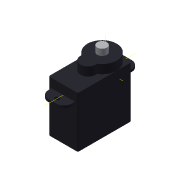
# Autodesk Inventor part: empty
Saved by Autodesk Inventor 2014 (Build 180170000, 170)
## iProperties
Created: 2015-04-13
Part Number: empty
Material: Generic
Document SubType Name: Modeling
Designer: Martin
Density: 1 g/cm^3
Appearance: Default
Author: Martin
Autodesk Inventor part; units mm, degrees
ref_plane "YZ Plane" through (0, 0, 0) normal (1, 0, 0) x (0, 1, 0)
ref_plane "XZ Plane" through (0, 0, 0) normal (0, 1, 0) x (-1, 0, 0)
ref_plane "XY Plane" through (0, 0, 0) normal (0, 0, 1) x (1, 0, 0)
sketch "Sketch1" plane through (0, 0, 0) normal (1, 0, 0) x (0, 1, 0)
  line L0 (0, -20.5) -> (0, 7.5) projected
  line L1 (-20.7, 0) -> (8.7, 0) projected
  line L2 (4.5, 3.5) -> (-16.5, 3.5)
  line L3 (-16.5, 3.5) -> (-16.5, -16.5)
  line L4 (-16.5, -16.5) -> (4.5, -16.5)
  line L5 (4.5, -16.5) -> (4.5, 3.5)
  point P0 (0, 0)
  dimension "d0" = 4.5
  dimension "d1" = 20
  dimension "d2" = 21
  dimension "d3" = 3.5
  constraints: 8 end point, 2 parallel, 1 horizontal, 1 perpendicular
  measures "d0" distance between parallel lines of L5 L0
  measures "d1" distance of L4.end L2.start
  measures "d2" distance of L3.end L4.end
  measures "d3" distance between parallel lines of L1 L2
extrude "Extrusion1" add sketch "Sketch1" along normal mid plane 11.5
sketch "Sketch2" plane through (0, 0, 0) normal (0, 0, 1) x (1, 0, 0)
  line L0 (5.75, 4.5) -> (-5.75, 4.5) projected
  line L1 (-5.75, 4.5) -> (5.75, 4.5) projected
  line L2 (-5.75, -16.5) -> (5.75, -16.5) projected
  line L3 (-5.75, -16.5) -> (5.75, -16.5) projected
  line L4 (-5.75, 4.5) -> (5.75, 4.5)
  line L5 (4.6, 8.8) -> (-4.6, 8.8)
  line L6 (-5.75, -16.5) -> (5.75, -16.5)
  circle A0 centre (0, 6.875) radius 0.925
  line L7 (0, -26.72) -> (0, 14.72) projected
  line L8 (-5.75, -16.5) -> (-5.75, 4.5) projected
  line L9 (5.75, 4.5) -> (5.75, -16.5) projected
  line L10 (-5.75, -6) -> (5.75, -6) construction
  circle A1 centre (0, -18.875) radius 0.925
  line L11 (-4.6, 8.8) -> (-4.6, 4.5)
  line L12 (4.6, 8.8) -> (4.6, 4.5)
  line L13 (-4.6, -16.5) -> (-4.6, -20.8)
  line L14 (-4.6, -20.8) -> (4.6, -20.8)
  line L15 (4.6, -20.8) -> (4.6, -16.5)
  point P0 (0, 0)
  point P1 (0, 7.8)
  dimension "d7" = 1.85
  dimension "d8" = 3.3
  dimension "d12" = 9.2
  dimension "d13" = 4.3
  constraints: 18 end point, 7 point on line, 4 parallel, 4 perpendicular, 2 midpoint, 1 centre point, 1 collinear, 1 vertical alignment, 7 other
  measures "d8" distance from line of L0 point (0, 7.8)
  measures "d12" distance between parallel lines of L12 L11
  measures "d13" distance between parallel lines of L0 L5
extrude "Extrusion2" add sketch "Sketch2" against normal blind 1 contours L0 L7 A0 L5 L12 | L0 L11 L5 L7 A0 | L15 L14 L7 A1 L2 | L7 A1 L14 L13 L2
fillet "Fillet1" radius 3 4 edges at (4.6, 8.8, -0.5) (-4.6, 8.8, -0.5) (-4.6, -20.8, -0.5) (4.6, -20.8, -0.5)
fillet "Fillet2" radius 0.5 4 edges at (5.75, -16.5, -6.5) (-5.75, -16.5, -6.5) (-5.75, 4.5, -6.5) (5.75, 4.5, -6.5)
sketch "Sketch3" plane through (-5.25, 4.5, 3.5) normal (0, 0, 1) x (1, 0, 0)
  line L0 (11, -0.5) -> (11, -20.5) projected
  line L1 (5.25, -5.75) -> (5.25, -11.25) construction
  circle A0 centre (5.25, -11.25) radius 3
  line L2 (10.5, 0) -> (0, 0) projected
  line L3 (-0.5, -20.5) -> (-0.5, -0.5) projected
  circle A1 centre (5.25, -5.75) radius 5.75
  point P0 (5.25, -4.5)
  dimension "d16" = 6
  dimension "d17" = 5.5
  constraints: 3 tangent, 2 centre point, 2 coincident, 2 end point, 1 parallel
  measures "d16" diameter of A0
  measures "d17" distance of L1.start L1.end
extrude "Extrusion3" add sketch "Sketch3" along normal blind 3.45
sketch "Sketch4" plane through (-5.25, 4.5, 6.95) normal (0, 0, 1) x (1, 0, 0)
  arc A0 (8.1968, -10.6875) -> (2.3032, -10.6875) centre (5.25, -5.75) ccw projected
  circle A1 centre (5.25, -5.75) radius 1.875
  point P0 (5.25, -4.5)
  dimension "d20" = 3.75
  constraints: 1 centre point, 1 coincident
  measures "d20" diameter of A1
extrude "Extrusion4" add sketch "Sketch4" along normal blind 2.45
body "Solid1"
